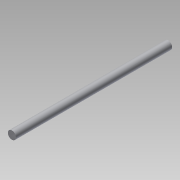
# Autodesk Inventor part: AWI-10
Saved by Autodesk Inventor 2020.1 (Build 241239000, 239)
## iProperties
Created: 2019-12-11
Part Number: AWI-10
Material: Aluminum-6061
Catalog Web Link: http://www.igus.com/WPCK/default.aspx?pagenr=5364&CL=US-en
Description: Drylin S Aluminum Shaft
Vendor: igus
Document SubType Name: Modeling
Mass: 163.494 g
Surface Area: 155.971 cm^2
Volume: 60.3299 cm^3
Density: 2.71 g/cm^3
Project: FIRST
Appearance: Aluminum - Flat
Designer: Autodesk, Inc.
Category: FIRST 2020 KOP
Company: Autodesk, Inc.
Title: Drylin S Aluminum Shaft
Author: Autodesk, Inc.
Autodesk Inventor part; units mm, degrees
ref_plane "YZ Plane" through (0, 0, 0) normal (1, 0, 0) x (0, 1, 0)
ref_plane "XZ Plane" through (0, 0, 0) normal (0, 1, 0) x (-1, 0, 0)
ref_plane "XY Plane" through (0, 0, 0) normal (0, 0, 1) x (1, 0, 0)
sketch "Sketch1" plane through (0, 0, 0) normal (0, 0, 1) x (1, 0, 0)
  circle A0 centre (0, 0) radius 7.9375
  dimension "d0" = 15.875
  constraints: 1 centre point, 1 coincident
  measures "d0" diameter of A0
extrude "Extrusion1" add sketch "Sketch1" along normal blind 304.8
body "Solid1"
